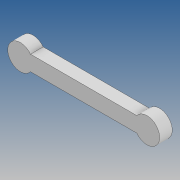
# Autodesk Inventor part: 2stopien
Saved by Autodesk Inventor 2022.3 (Build 263350000, 350)
## iProperties
Created: 2023-06-25
Part Number: 2stopien
Material: Ogólny
Document SubType Name: Modeling
Designer: Chyba Ja
Density: 1 g/cm^3
Appearance: Domyślna
Author: Chyba Ja
Autodesk Inventor part; units mm, degrees
ref_plane "YZ Plane" through (0, 0, 0) normal (1, 0, 0) x (0, 1, 0)
ref_plane "XZ Plane" through (0, 0, 0) normal (0, 1, 0) x (-1, 0, 0)
ref_plane "XY Plane" through (0, 0, 0) normal (0, 0, 1) x (1, 0, 0)
sketch "Szkic1" plane through (0, 0, 0) normal (0, 0, 1) x (1, 0, 0)
  arc A0 (20, 15) -> (-20, 15) centre (0, 0) ccw
  line L0 (20, 15) -> (125, 15)
  line L1 (125, 15) -> (125, -15)
  line L2 (125, -15) -> (20, -15)
  arc A1 (230, -15) -> (230, 15) centre (250, 0) ccw
  line L3 (230, 15) -> (125, 15)
  line L4 (125, -15) -> (230, -15)
  arc A2 (-20, 15) -> (20, -15) centre (0, 0) ccw
  dimension "d0" = 50
  dimension "d1" = 30
  dimension "d2" = 250
  constraints: 10 end point, 6 point on circle, 5 symmetric about line, 4 coincident, 3 centre point, 1 horizontal, 1 parallel, 1 perpendicular, 1 point on line, 1 vertical alignment, 1 other
  measures "d0" diameter of A0
  measures "d1" distance between parallel lines of L2 L0
  measures "d2" distance of point (0, 0) point (250, 0)
extrude "Wyciągnięcie proste1" add sketch "Szkic1" along normal blind 25
